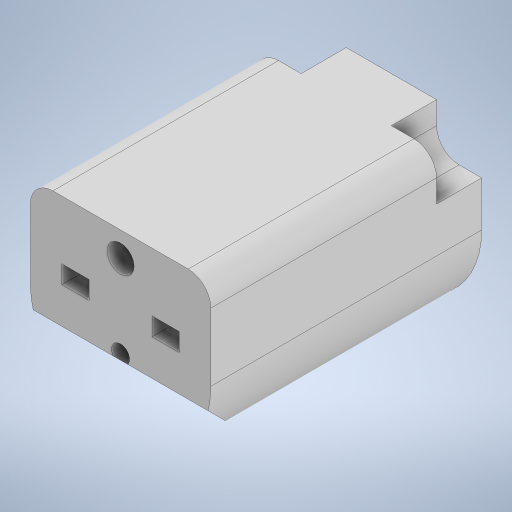
# Autodesk Inventor part: Fingertip Midpart
Saved by Autodesk Inventor 2023 (Build 270158000, 158)
## iProperties
Created: 2023-04-05
Part Number: Fingertip Midpart
Material: Generic
Document SubType Name: Modeling
Designer: 1roweste
Density: 1 g/cm^3
Appearance: Default
Author: 1roweste
Autodesk Inventor part; units mm, degrees
ref_plane "YZ Plane" through (0, 0, 0) normal (1, 0, 0) x (0, 1, 0)
ref_plane "XZ Plane" through (0, 0, 0) normal (0, 1, 0) x (-1, 0, 0)
ref_plane "XY Plane" through (0, 0, 0) normal (0, 0, 1) x (1, 0, 0)
sketch "Finger Body" plane through (0, 0, 0) normal (0, 0, 1) x (1, 0, 0)
  line L0 (-10, 10) -> (10, 10)
  line L1 (10, 10) -> (10, -10)
  line L2 (10, -10) -> (-10, -10)
  line L3 (-10, -10) -> (-10, 10)
  arc A0 (-10, 0) -> (10, 0) centre (0, 0) ccw
  line L4 (-10, 0) -> (10, 0)
  circle A1 centre (-7.5, 7.5) radius 2.5
  circle A2 centre (7.5, 7.5) radius 2.5
  circle A3 centre (0, 0) radius 8.75
  line L5 (0, -8.75) -> (1, -8.75) construction
  line L6 (1, 8.6927) -> (1, -8.75)
  line L7 (-1, 8.6927) -> (-1, -8.6927)
  line L8 (-1, -9.9499) -> (-1, -10)
  circle A4 centre (0, 7.25) radius 1.5
  circle A5 centre (0, -1.929) radius 1
  point P0 (1, -8.6927)
  point P1 (10, 7.5)
  point P2 (7.5, 10)
  point P3 (-7.5, 10)
  point P4 (-10, 7.5)
  dimension "d0" = 20
  dimension "d1" = 20
  dimension "d2" = 10
  dimension "d3" = 10
  dimension "d4" = 5
  dimension "d5" = 2.5
  dimension "d6" = 2.5
  dimension "d7" = 5
  dimension "d8" = 2.5
  dimension "d9" = 2.5
  dimension "d10" = 17.5
  dimension "d42" = 3
  dimension "d43" = 0
  dimension "d44" = 0
  dimension "d45" = 9.179
  dimension "d46" = 0
  constraints: 18 end point, 7 point on circle, 6 centre point, 2 coincident, 2 horizontal, 2 midpoint, 2 parallel, 1 perpendicular, 1 tangent
  measures "d0" distance of L1.end L2.end
  measures "d1" distance of L0.end L1.end
  measures "d2" distance from line of point (0, 0) L3
  measures "d3" distance from line of L0 point (0, 0)
  measures "d4" diameter of A1
  measures "d5" distance from line of L3 A1.centre
  measures "d6" distance from line of L0 A1.centre
  measures "d7" diameter of A2
  measures "d8" distance from line of L1 A2.centre
  measures "d9" distance from line of L0 A2.centre
  measures "d10" diameter of A3
  measures "d42" diameter of A4
  measures "d43" horizontal distance of A3.centre A4.centre
  measures "d44" horizontal distance between centres of A3 A4
  measures "d45" distance of A4.centre A5.centre
  measures "d46" horizontal distance of A4.centre A5.centre
sketch "Cap Imprint (DNE)" plane through (0, 0, 0) normal (0, 0, 1) x (1, 0, 0)
  circle A0 centre (0, 0) radius 8.75 projected
  arc A1 (-10, 0) -> (10, 0) centre (0, 0) ccw projected
  line L0 (-10, -10) -> (-10, 10) projected
  line L1 (-10, 10) -> (10, 10) projected
  line L2 (10, 10) -> (10, -10) projected
  line L3 (1, 8.6927) -> (1, -8.75) projected
  line L4 (-1, 8.6927) -> (-1, -8.6927) projected
  circle A2 centre (-7.5, 7.5) radius 2.5 projected
  circle A3 centre (7.5, 7.5) radius 2.5 projected
  circle A4 centre (0, 0) radius 0.5
  dimension "d15" = 1
  constraints: 1 centre point, 1 coincident
  measures "d15" diameter of A4
extrude "FingerLength (Scale for each finger)" add sketch "Finger Body" along normal blind 30 contours L0 A2 A3 A1 | A1 A3 | A1 A3 L4 L3 | A2 A3 | L4 A3 A0 | A3 A1 | A1 A3 L7 A4 L4 | L1 L4 A3 A2 | A3 A2 | A2 A3 L4 L6 A4 | L4 L7 A3 | L6 A4 A3 | A3 A4 L7 | L7 A4 L6 L4 | L4 L6 A5 L7 | L7 A5 L6 A3 | A3 L6 L4
sketch "Sketch3" plane through (0, 0, 30) normal (0, 0, 1) x (1, 0, 0)
  arc A0 (-7.5, 10) -> (-10, 7.5) centre (-7.5, 7.5) ccw projected
  line L0 (-10, 7.5) -> (-7, 7.5)
  line L1 (-7, 7.5) -> (-6.5, 7.5)
  line L2 (-6.5, 7.5) -> (-3.5, 7.5)
  line L3 (-3.5, 7.5) -> (-3, 7.5)
  arc A1 (10, 7.5) -> (7.5, 10) centre (7.5, 7.5) ccw projected
  line L4 (10, 7.5) -> (7, 7.5)
  line L5 (7, 7.5) -> (6.5, 7.5)
  line L6 (6.5, 7.5) -> (3.5, 7.5)
  line L7 (3.5, 7.5) -> (3, 7.5)
  line L8 (-6.5, 7.5) -> (-3.5, 7.5)
  line L9 (-3.5, 7.5) -> (-3.5, -2.5)
  line L10 (-3.5, -2.5) -> (-6.5, -2.5)
  line L11 (-6.5, -2.5) -> (-6.5, 7.5)
  line L12 (6.5, 7.5) -> (3.5, 7.5)
  line L13 (3.5, 7.5) -> (3.5, -2.5)
  line L14 (3.5, -2.5) -> (6.5, -2.5)
  line L15 (6.5, -2.5) -> (6.5, 7.5)
  line L16 (-6.5, 2.5) -> (6.5, 2.5)
  line L17 (-6.5, 3.5) -> (6.5, 3.5)
  line L18 (-6.5, 1.5) -> (6.5, 1.5)
  point P0 (0, 0)
  point P1 (-3.5, 1.5)
  point P2 (-3.5, 3.5)
  point P3 (3.5, 1.5)
  point P4 (3.5, 3.5)
  dimension "d18" = 3
  dimension "d19" = 0.5
  dimension "d20" = 3
  dimension "d21" = 0.5
  dimension "d22" = 3
  dimension "d23" = 0.5
  dimension "d24" = 3
  dimension "d25" = 0.5
  dimension "d26" = 10
  dimension "d27" = 10
  dimension "d28" = 1
  dimension "d29" = 1
  constraints: 38 end point, 6 parallel, 6 point on line, 4 horizontal, 2 midpoint, 2 perpendicular
  measures "d18" distance of L0.start L0.end
  measures "d19" distance of L0.end L1.end
  measures "d20" distance of L1.end L2.end
  measures "d21" distance of L2.end L3.end
  measures "d22" distance of L4.start L4.end
  measures "d23" distance of L4.end L5.end
  measures "d24" distance of L5.end L6.end
  measures "d25" distance of L6.end L7.end
  measures "d26" distance of L8.end L9.end
  measures "d27" distance of L13.end L12.end
  measures "d28" distance between parallel lines of L16 L17
  measures "d29" distance between parallel lines of L16 L18
extrude "Extrusion2" cut sketch "Sketch3" against normal blind 4 contours L17 L9 L16 L11 | L16 L9 L18 L11 | L17 L15 L16 L13 | L16 L15 L18 L13
sketch "Sketch4" plane through (10, 0, 0) normal (1, 0, 0) x (0, 0, -1)
  line L0 (0, -10) -> (-30, -10) projected
  line L1 (-30, 0) -> (-30, -10) projected
  line L2 (-30, 0) -> (-30, 7.5) projected
  line L3 (-30, 10) -> (-30, 7.5) projected
  line L4 (0, 10) -> (-30, 10) projected
  line L5 (0, 0) -> (0, 7.5) projected
  line L6 (0, 10) -> (0, 7.5) projected
  line L7 (0, 0) -> (0, -10) projected
  line L8 (0, 7.5) -> (-30, 7.5) projected
  line L9 (-30, 7.5) -> (-30, -2.5)
  line L10 (-30, -8.6927) -> (-30, 8.6927) projected
  line L11 (-30, -2.5) -> (-22.5, -10)
  dimension "d32" = 10
  dimension "d33" = 135
  constraints: 4 end point, 2 point on line
  measures "d32" distance of L2.end L9.end
  measures "d33" angle of L11 L9
extrude "Extrusion3" cut sketch "Sketch4" against normal up to surface (20 mm away) contours L0 L1 L11
sketch "Sketch5" plane through (0, 0, 0) normal (0, 0, -1) x (-1, 0, 0)
  arc A0 (-7.5, 10) -> (-10, 7.5) centre (-7.5, 7.5) ccw projected
  line L0 (-10, 0) -> (-10, 7.5) projected
  arc A1 (-10, 0) -> (10, 0) centre (0, 0) ccw projected
  line L1 (10, 7.5) -> (10, 0) projected
  arc A2 (10, 7.5) -> (7.5, 10) centre (7.5, 7.5) ccw projected
  line L2 (-7.5, 10) -> (7.5, 10) projected
  circle A3 centre (-7.5, 7.5) radius 2.5
  circle A4 centre (7.5, 7.5) radius 2.5
  line L3 (-7.5, 5) -> (-10, 5)
  line L4 (-10, 0) -> (-10, 7.5) projected
  line L5 (7.5, 5) -> (10, 5)
  line L6 (-5, 7.5) -> (-5, 10)
  line L7 (5, 7.5) -> (5, 10)
  line L8 (-1, -8.6927) -> (-1, -9.9499)
  line L9 (1, -8.6927) -> (1, -9.9499)
  line L10 (-2, -8.6927) -> (-2, -9.9499)
  line L11 (-3.5, -8.6927) -> (-3.5, -9.9499)
  line L12 (2, -8.6927) -> (2, -9.9499)
  line L13 (3.5, -8.6927) -> (3.5, -9.9499)
  line L14 (-3.5, -8.6927) -> (-2, -8.6927)
  line L15 (2, -8.6927) -> (3.5, -8.6927)
  point P0 (2, -9.798)
  point P1 (3.5, -9.3675)
  point P2 (-3.5, -9.3675)
  point P3 (-2, -9.798)
  dimension "d38" = 1
  dimension "d39" = 1.5
  dimension "d40" = 1
  dimension "d41" = 1.5
  constraints: 24 end point, 6 point on circle, 5 equal length, 4 perpendicular, 4 point on line, 2 centre point, 2 coincident, 2 tangent, 1 horizontal, 1 vertical
  measures "d38" distance between parallel lines of L8 L10
  measures "d39" distance between parallel lines of L10 L11
  measures "d40" distance between parallel lines of L9 L12
  measures "d41" distance between parallel lines of L12 L13
extrude "Extrusion4" cut sketch "Sketch5" against normal blind 5 contours A3 A0 | L2 L6 A3 | A3 L3 L0 | L2 A4 L7 | A2 A4 | L11 L14 L10 A1 | L1 L5 A4 | A1 L12 L15 L13
sketch "End Imprint (DNE)" plane through (0, 0, 0) normal (0, 0, -1) x (-1, 0, 0)
  line L0 (-5, 10) -> (-5, 7.5) projected
  arc A0 (-7.5, 5) -> (-5, 7.5) centre (-7.5, 7.5) ccw projected
  line L1 (-7.5, 5) -> (-10, 5) projected
  line L2 (-10, 0) -> (-10, 5) projected
  arc A1 (-10, 0) -> (-3.5, -9.3675) centre (0, 0) ccw projected
  line L3 (-3.5, -9.3675) -> (-3.5, -8.6927) projected
  line L4 (-3.5, -8.6927) -> (-2, -8.6927) projected
  line L5 (-2, -8.6927) -> (-2, -9.798) projected
  arc A2 (-2, -9.798) -> (2, -9.798) centre (0, 0) ccw projected
  line L6 (2, -9.798) -> (2, -8.6927) projected
  line L7 (2, -8.6927) -> (3.5, -8.6927) projected
  line L8 (3.5, -8.6927) -> (3.5, -9.3675) projected
  arc A3 (3.5, -9.3675) -> (10, 0) centre (0, 0) ccw projected
  line L9 (10, 5) -> (10, 0) projected
  line L10 (10, 5) -> (7.5, 5) projected
  arc A4 (5, 7.5) -> (7.5, 5) centre (7.5, 7.5) ccw projected
  line L11 (5, 7.5) -> (5, 10) projected
  line L12 (-5, 10) -> (5, 10) projected
  arc A5 (-7.5, 5) -> (-5, 7.5) centre (-7.5, 7.5) ccw projected
  line L13 (-5, 10) -> (-5, 7.5) projected
  line L14 (-7.5, 10) -> (-5, 10) projected
  arc A6 (-7.5, 10) -> (-10, 7.5) centre (-7.5, 7.5) ccw projected
  line L15 (-10, 5) -> (-10, 7.5) projected
  line L16 (-7.5, 5) -> (-10, 5) projected
  arc A7 (10, 7.5) -> (7.5, 10) centre (7.5, 7.5) ccw projected
  line L17 (5, 10) -> (7.5, 10) projected
  line L18 (5, 7.5) -> (5, 10) projected
  arc A8 (5, 7.5) -> (7.5, 5) centre (7.5, 7.5) ccw projected
  line L19 (10, 5) -> (7.5, 5) projected
  line L20 (10, 7.5) -> (10, 5) projected
  line L21 (2, -9.798) -> (2, -8.6927) projected
  arc A9 (2, -9.798) -> (3.5, -9.3675) centre (0, 0) ccw projected
  line L22 (3.5, -8.6927) -> (3.5, -9.3675) projected
  line L23 (2, -8.6927) -> (3.5, -8.6927) projected
  line L24 (-3.5, -9.3675) -> (-3.5, -8.6927) projected
  arc A10 (-3.5, -9.3675) -> (-2, -9.798) centre (0, 0) ccw projected
  line L25 (-2, -8.6927) -> (-2, -9.798) projected
  line L26 (-3.5, -8.6927) -> (-2, -8.6927) projected
body "Solid1"
